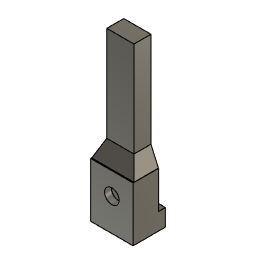
SolderingStation_TransfoSupport (Autodesk Fusion 360 design; units mm, degrees)
Autodesk Fusion 360 part; units mm, degrees
sketch "Sketch1" plane through (0, 0, 0) normal (0, 0, 1) x (1, 0, 0)
  line L0 (4.25, 2.75) -> (-4.25, 2.75)
  line L1 (-4.25, 2.75) -> (-4.25, -2.75)
  line L2 (-4.25, -2.75) -> (4.25, -2.75)
  line L3 (4.25, -2.75) -> (4.25, 2.75)
  line L4 (4.25, 2.75) -> (-4.25, -2.75) construction
  line L5 (-4.25, 2.75) -> (4.25, -2.75) construction
  line L6 (-6.25, -4.75) -> (6.25, -4.75)
  line L7 (6.25, -4.75) -> (6.25, 4.75)
  line L8 (6.25, 4.75) -> (-6.25, 4.75)
  line L9 (-6.25, 4.75) -> (-6.25, -4.75)
  line L10 (-4.25, 2.75) -> (-6.25, 2.75)
  line L11 (4.25, 2.75) -> (6.25, 2.75)
  dimension "d1" = 8.5
  dimension "d2" = 5.5
  dimension "d3" = 2
  constraint horizontal L0
  constraint perpendicular L0 L1
  constraint parallel L0 L2
  constraint parallel L1 L3
  constraint coincident L4 origin
  constraint coincident L5 origin
  constraint coincident L9 L10.end
  constraint perpendicular L9 L10
  constraint coincident L7 L11.end
  constraint perpendicular L7 L11
  measures "d1" distance of L1.end L2.end
  measures "d2" distance of L0.end L1.end
extrude "Extrude1" add sketch "Sketch1" along normal blind 8.2 contours L1 L2 L3 L6 L7 L9 L10 L11
sketch "Sketch2" plane through (0, 0, 8.2) normal (0, 0, 1) x (-1, 0, 0)
  line L0 (4.25, -2.75) -> (6.25, -2.75)
  line L1 (6.25, -2.75) -> (6.25, 4.75)
  line L2 (6.25, 4.75) -> (-6.25, 4.75)
  line L3 (-6.25, 4.75) -> (-6.25, -2.75)
  line L4 (-6.25, -2.75) -> (-4.25, -2.75)
  line L5 (-4.25, -2.75) -> (-4.25, 2.75)
  line L6 (-4.25, 2.75) -> (4.25, 2.75)
  line L7 (4.25, 2.75) -> (4.25, -2.75)
  line L8 (6.25, -2.75) -> (-6.25, -2.75)
  line L9 (-6.25, -2.75) -> (-6.25, 4.75)
  line L10 (-6.25, 4.75) -> (6.25, 4.75)
  line L11 (6.25, 4.75) -> (6.25, -2.75)
  constraint horizontal L8
  constraint vertical L9
  constraint horizontal L10
  constraint vertical L11
  constraint coincident L2.end L3.start
  constraint coincident L0.end L1.start
extrude "Extrude2" add sketch "Sketch2" along normal blind 2
sketch "Sketch4" plane through (0, 0, 10.2) normal (0, 0, 1) x (-1, 0, 0)
  line L0 (6.25, 4.75) -> (-6.25, 4.75)
  line L1 (-6.25, 4.75) -> (-6.25, -2.75)
  line L2 (-6.25, -2.75) -> (6.25, -2.75)
  line L3 (6.25, -2.75) -> (6.25, 4.75)
  line L4 (4, -2.75) -> (-4, -2.75)
  line L5 (-4, -2.75) -> (-4, 2.25)
  line L6 (-4, 2.25) -> (4, 2.25)
  line L7 (4, 2.25) -> (4, -2.75)
  line L8 (0, -2.75) -> (0, 4.75) construction
  dimension "d8" = 8
  dimension "d9" = 5
  dimension "d10" = 4
  constraint horizontal L4
  constraint vertical L5
  constraint horizontal L6
  constraint vertical L7
  constraint coincident L2 L4.start
  constraint midpoint L2 L8.start
  constraint midpoint L0 L8.end
  measures "d8" distance of L4.start L4.end
  measures "d9" distance of L4.end L5.end
  measures "d10" distance of L7 L8
extrude "Extrude3" add sketch "Sketch4" along normal blind 43 contours L2 L4 L5 L6 L7
sketch "Sketch5" plane through (0, -4.75, 0) normal (0, -1, 0) x (1, 0, 0)
  line L0 (-6.25, 0) -> (6.25, 0)
  line L1 (6.25, 0) -> (6.25, 10.2)
  line L2 (6.25, 10.2) -> (-6.25, 10.2)
  line L3 (-6.25, 10.2) -> (-6.25, 0)
  circle A0 centre (0, 3.7) radius 2.15
  line L4 (-4.25, 8.2) -> (4.25, 8.2)
  dimension "d13" = 4.3
  dimension "d18" = 4.5
  measures "d13" diameter of A0
  measures "d18" distance of A0.centre L4
extrude "Extrude4" cut sketch "Sketch5" against normal blind 2 contours A0
chamfer "Chamfer1" distance 2.2 distance2 5 3 edges at (0, -2.25, 10.2) (4, 0.25, 10.2) (-4, 0.25, 10.2) measured on face at (-1.3333, -3.9167, 10.2) measured on face at (-1.3333, -3.9167, 10.2) measured on face at (-1.3333, -3.9167, 10.2)
extrude "Extrude5" add 1 faces at (-1.4167, -4.0833, 0) along direction (0, 0, -1) blind 0.8
extrude "Extrude6" add 1 faces at (-1.4167, -4.0833, -0.8) along direction (0, 0, -1) blind 5
sketch "Sketch6" plane through (0, 2.75, 0) normal (0, 1, 0) x (-1, 0, 0)
  line L0 (6.25, -5.8) -> (6.25, 10.2)
  line L1 (6.25, 10.2) -> (6.2, 10.2)
  line L2 (6.2, 10.2) -> (4, 15.2)
  line L3 (4, 15.2) -> (4, 53.2)
  line L4 (4, 53.2) -> (-4, 53.2)
  line L5 (-4, 53.2) -> (-4, 15.2)
  line L6 (-4, 15.2) -> (-6.2, 10.2)
  line L7 (-6.2, 10.2) -> (-6.25, 10.2)
  line L8 (-6.25, 10.2) -> (-6.25, -5.8)
  line L9 (-6.25, -5.8) -> (-4.25, -5.8)
  line L10 (-4.25, -5.8) -> (-4.25, 8.2)
  line L11 (-4.25, 8.2) -> (4.25, 8.2)
  line L12 (4.25, 8.2) -> (4.25, -5.8)
  line L13 (4.25, -5.8) -> (6.25, -5.8)
  line L14 (-6.25, -5.8) -> (6.25, -5.8)
  line L15 (6.25, -5.8) -> (6.25, -0.8)
  line L16 (6.25, -0.8) -> (-6.25, -0.8)
  line L17 (-6.25, -0.8) -> (-6.25, -5.8)
  dimension "d23" = 5
  dimension "d28" = 12.5
  constraint horizontal L14
  constraint vertical L15
  constraint horizontal L16
  constraint vertical L17
  constraint coincident L8.end L9.start
  measures "d23" distance of L8.end L16.end
  measures "d28" distance of L8.end L0.start
extrude "Extrude7" add sketch "Sketch6" along normal blind 2 contours L0 L12 L13 L14 L15 L16 | L10 L12 L14 L16 | L8 L9 L10 L14 L16 L17
extrude "Extrude8" cut 1 faces at (1.3333, 1.0833, 53.2) along direction (0, 0, -1) blind 10
equation "d18 = 2.35 mm + 2.15 mm"
